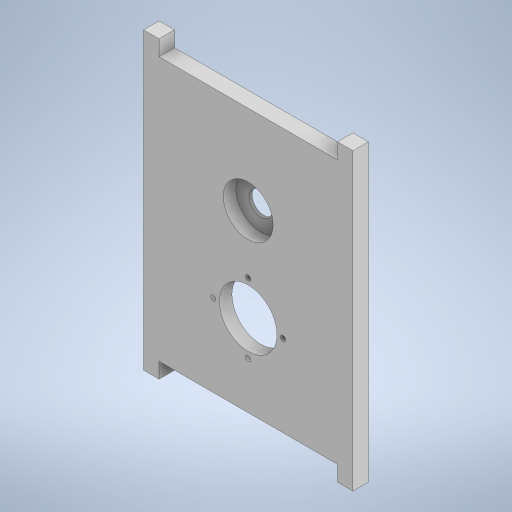
# Autodesk Inventor part: side1
Saved by Autodesk Inventor 2023 (Build 270158000, 158)
## iProperties
Created: 2023-05-27
Part Number: side1
Material: 一般
Document SubType Name: Modeling
Designer: 310611102
Density: 1 g/cm^3
Appearance: 預設
Author: 310611102
Autodesk Inventor part; units mm, degrees
ref_plane "YZ Plane" through (0, 0, 0) normal (1, 0, 0) x (0, 1, 0)
ref_plane "XZ Plane" through (0, 0, 0) normal (0, 1, 0) x (-1, 0, 0)
ref_plane "XY Plane" through (0, 0, 0) normal (0, 0, 1) x (1, 0, 0)
sketch "Sketch1" plane through (0, 0, 0) normal (0, 0, 1) x (1, 0, 0)
  line L0 (-57.5, 85) -> (57.5, 85)
  line L1 (67.5, 45.4637) -> (67.5, -85)
  line L2 (57.5, -85) -> (-57.5, -85)
  line L3 (-67.5, -45.4637) -> (-67.5, 85)
  line L4 (-67.5, 85) -> (67.5, -85) construction
  line L5 (67.5, 45.4637) -> (-67.5, -45.4637) construction
  line L6 (-57.5, 95) -> (-67.5, 95)
  line L7 (-67.5, 95) -> (-67.5, 85)
  line L8 (-57.5, 85) -> (-57.5, 95)
  line L9 (-57.5, 95) -> (-67.5, 85) construction
  line L10 (-67.5, 95) -> (-57.5, 85) construction
  line L11 (0, 15.2738) -> (0, -11.5274)
  line L12 (-10.8069, 0) -> (18.2997, 0)
  line L13 (57.5, 95) -> (67.5, 95)
  line L14 (67.5, 95) -> (67.5, 45.4637)
  line L15 (57.5, 85) -> (57.5, 95)
  line L16 (57.5, 95) -> (67.5, 45.4637) construction
  line L17 (67.5, 95) -> (57.5, 85) construction
  line L18 (-57.5, -95) -> (-67.5, -95)
  line L19 (-67.5, -95) -> (-67.5, -45.4637)
  line L20 (-57.5, -85) -> (-57.5, -95)
  line L21 (-57.5, -95) -> (-67.5, -45.4637) construction
  line L22 (-67.5, -95) -> (-57.5, -85) construction
  line L23 (57.5, -95) -> (67.5, -95)
  line L24 (67.5, -95) -> (67.5, -85)
  line L25 (57.5, -85) -> (57.5, -95)
  line L26 (57.5, -95) -> (67.5, -85) construction
  line L27 (67.5, -95) -> (57.5, -85) construction
  point P0 (0, 0)
  point P1 (-62.5, 90)
  point P2 (62.5, 90)
  point P3 (-62.5, -90)
  point P4 (62.5, -90)
  dimension "d0" = 135
  dimension "d1" = 10
  dimension "d2" = 170
  constraints: 52 end point, 12 symmetric about line, 4 midpoint, 3 horizontal, 3 parallel, 3 perpendicular, 2 point on line, 1 vertical, 6 other
  measures "d0" distance between parallel lines of L3 L1
  measures "d1" distance of L6.start L6.end
  measures "d2" distance between parallel lines of L2 L0
extrude "Extrusion1" add sketch "Sketch1" along normal blind 10
sketch "Sketch2" plane through (0, 0, 10) normal (0, 0, 1) x (1, 0, 0)
  circle A0 centre (0, 27.8) radius 16
  circle A1 centre (0, -32.2) radius 18.5
  line L0 (-57.5, -85) -> (57.5, -85) projected
  point P0 (0, 0)
  dimension "d6" = 32
  dimension "d11" = 37
  dimension "d14" = 52.8
  dimension "d15" = 60
  constraints: 2 centre point, 2 vertical alignment, 1 other
  measures "d6" diameter of A0
  measures "d11" diameter of A1
  measures "d14" distance from line of L0 A1.centre
  measures "d15" distance of A1.centre A0.centre
extrude "Extrusion2" cut sketch "Sketch2" against normal blind 8
sketch "Sketch3" plane through (0, 27.8, 2) normal (0, 0, 1) x (1, 0, 0)
  circle A0 centre (0, 0) radius 7.5
  circle A1 centre (0, 0) radius 16 projected
  point P0 (0, -27.8)
  dimension "d16" = 15
  constraints: 1 centre point, 1 concentric
  measures "d16" diameter of A0
extrude "Extrusion3" cut sketch "Sketch3" against normal through all contours A0
sketch "Sketch6" plane through (0, -32.2, 2) normal (0, 0, 1) x (1, 0, 0)
  circle A0 centre (0, 0) radius 25
  point P0 (0, 32.2)
  dimension "d19" = 50
  constraints: 1 centre point
  measures "d19" diameter of A0
extrude "Extrusion4" cut sketch "Sketch6" against normal blind 10
sketch "Sketch7" plane through (0, -32.2, 2) normal (0, 0, -1) x (-1, 0, 0)
  circle A0 centre (0, 22.5) radius 1.6
  circle A1 centre (-22.5, 0) radius 1.6
  circle A2 centre (0, -22.5) radius 1.6
  circle A3 centre (22.5, 0) radius 1.6
  point P0 (0, 32.2)
  point P1 (0, 0)
  dimension "d22" = 3.2
  dimension "d25" = 360
  dimension "d27" = 45
  constraints: 4 centre point, 1 vertical alignment, 10 other
  measures "d22" diameter of A0
  measures "d27" distance of A2.centre A0.centre
extrude "Extrusion5" cut sketch "Sketch7" against normal blind 10
body "Solid1"
